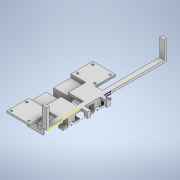
# Autodesk Inventor part: shell 1.0 screw
Saved by Autodesk Inventor 2020.2 (Build 242310000, 310)
## iProperties
Created: 2020-02-28
Part Number: shell 1.0 screw
Material: Generic
Document SubType Name: Modeling
Designer: ColinP
Density: 1 g/cm^3
Appearance: Default
Author: ColinP
Autodesk Inventor part; units mm, degrees
ref_plane "YZ Plane" through (0, 0, 0) normal (1, 0, 0) x (0, 1, 0)
ref_plane "XZ Plane" through (0, 0, 0) normal (0, 1, 0) x (-1, 0, 0)
ref_plane "XY Plane" through (0, 0, 0) normal (0, 0, 1) x (1, 0, 0)
sketch "Sketch1" plane through (0, 0, 0) normal (0, 1, 0) x (-1, 0, 0)
  line L0 (0, 0) -> (8, 0)
  line L1 (8, 0) -> (8, 116.7892)
  line L2 (8, 116.7892) -> (0, 116.7892)
  line L3 (0, 116.7892) -> (0, 0)
  line L4 (8, 0) -> (0, 0)
  line L5 (0, 0) -> (0, -4)
  line L6 (0, -4) -> (8, -4)
  line L7 (8, -4) -> (8, 0)
  line L8 (8, 116.7892) -> (0, 116.7892)
  line L9 (0, 116.7892) -> (0, 120.7892)
  line L10 (0, 120.7892) -> (8, 120.7892)
  line L11 (8, 120.7892) -> (8, 116.7892)
  point P0 (0, 116.7892)
  dimension "d0" = 8
  dimension "d1" = 116.7892
  dimension "d2" = 8
  dimension "d3" = 4
  dimension "d4" = 4
  constraints: 24 end point, 6 parallel, 3 horizontal, 3 perpendicular
  measures "d0" distance of L2.end L1.end
  measures "d1" distance of L1.end L0.end
  measures "d2" distance of L6.end L5.end
  measures "d3" distance of L5.end L4.end
  measures "d4" distance of L8.end L9.end
extrude "Extrusion1" add sketch "Sketch1" along normal blind 4 contours L3 L2 L1 L0
extrude "Extrusion2" add sketch "Sketch1" along normal blind 34 contours L0 L7 L6 L5 | L9 L10 L11 L2
sketch "Sketch2" plane through (0, 0, 0) normal (0, -1, 0) x (1, 0, 0)
  line L0 (0, 0) -> (0, 19.558)
  line L1 (0, 116.7892) -> (0, 0) projected
  line L2 (0, 19.558) -> (0, 35.6705)
  line L3 (0, 35.6705) -> (0, 48.3705)
  line L4 (0, 48.3705) -> (-8, 48.3705)
  line L5 (-8, 0) -> (-8, 116.7892) projected
  line L6 (-8, 19.558) -> (-8, 48.3705)
  line L7 (0, 19.558) -> (-8, 19.558)
  dimension "d9" = 19.558
  dimension "d10" = 16.1125
  dimension "d11" = 12.7
  constraints: 12 end point, 5 point on line, 2 perpendicular, 1 collinear
  measures "d9" distance of L0.start L0.end
  measures "d10" distance of L0.end L2.end
  measures "d11" distance of L2.end L3.end
extrude "Extrusion3" add sketch "Sketch2" along normal blind 25
sketch "Sketch3" plane through (0, 0, -4) normal (1, 0, 0) x (0, 0, -1)
  line L0 (-52.3705, -25) -> (-23.558, -25) projected
  line L1 (-37.9642, -25) -> (-37.9642, -13.8875)
  line L2 (-37.9642, -13.8875) -> (-31.5508, -13.8875)
  line L3 (-31.5508, -13.8875) -> (-44.3778, -13.8875)
  line L4 (-44.3778, -13.8875) -> (-41.1646, -8.3222)
  line L5 (-44.3778, -13.8875) -> (-37.9516, -13.8875) construction
  line L6 (-41.1646, -8.3222) -> (-34.7385, -8.3222)
  line L7 (-34.7385, -8.3222) -> (-31.5253, -13.8875)
  line L8 (-31.5253, -13.8875) -> (-34.7385, -19.4528)
  line L9 (-34.7385, -19.4528) -> (-41.1646, -19.4528)
  line L10 (-41.1646, -19.4528) -> (-44.3778, -13.8875)
  line L11 (-23.558, 0) -> (-23.558, -25) projected
  line L12 (-52.3705, 0) -> (-52.3705, -25) projected
  line L13 (-23.558, -25) -> (-52.3705, -25)
  line L14 (-52.3705, -25) -> (-52.3705, -13.8875)
  line L15 (-52.3705, -13.8875) -> (-23.558, -13.8875)
  line L16 (-23.558, -13.8875) -> (-23.558, -25)
  point P0 (-4, 0)
  point P1 (-23.558, -13.8875)
  point P2 (-31.5253, -13.8875)
  point P3 (-44.3778, -13.8875)
  dimension "d14" = 11.1125
  dimension "d15" = 6.4135
  dimension "d16" = 12.827
  dimension "d17" = 6.4262
  dimension "d18" = 60
  dimension "d19" = 6.4262
  dimension "d20" = 120
  dimension "d21" = 120
  dimension "d22" = 6.4262
  dimension "d23" = 120
  dimension "d24" = 6.4262
  dimension "d25" = 120
  constraints: 28 end point, 5 horizontal, 4 parallel, 2 point on line, 1 equal length, 1 midpoint, 1 perpendicular, 1 vertical
  measures "d14" distance of L1.start L1.end
  measures "d15" distance of L1.end L2.end
  measures "d16" distance of L2.end L3.end
  measures "d17" distance of L3.end L4.end
  measures "d18" angle of L5 L4
  measures "d19" distance of L4.end L6.end
  measures "d20" angle of L4 L6
  measures "d21" angle of L6 L7
  measures "d22" distance of L7.end L8.end
  measures "d23" angle of L7 L8
  measures "d24" distance of L8.end L9.end
  measures "d25" angle of L8 L9
extrude "Extrusion4" cut sketch "Sketch3" against normal blind 25.4
sketch "Sketch4" plane through (0, 0, -4) normal (1, 0, 0) x (0, 0, -1)
  line L0 (0, 0) -> (-23.558, 0) projected
  line L1 (-23.558, 0) -> (-29.558, 0)
  line L2 (-29.558, 0) -> (-29.558, -8.89)
  line L3 (-29.558, -8.89) -> (-23.558, -8.89)
  line L4 (-23.558, -8.89) -> (-23.558, 0)
  line L5 (-52.3705, 0) -> (-52.3705, -13.8875) projected
  line L6 (-52.3705, 0) -> (-46.3761, 0)
  line L7 (-46.3761, 0) -> (-46.3761, -8.89)
  line L8 (-46.3761, -8.89) -> (-52.3705, -8.89)
  line L9 (-52.3705, -8.89) -> (-52.3705, 0)
  point P0 (-4, 0)
  dimension "d28" = 6
  dimension "d29" = 8.89
  dimension "d30" = 5.9944
  dimension "d31" = 8.89
  constraints: 16 end point, 4 parallel, 2 horizontal, 2 perpendicular
  measures "d28" distance of L3.end L2.end
  measures "d29" distance of L2.end L1.end
  measures "d30" distance of L7.end L8.end
  measures "d31" distance of L6.end L7.end
extrude "Extrusion5" cut sketch "Sketch4" against normal blind 25.4
sketch "Sketch6" plane through (0, 0, -4) normal (1, 0, 0) x (0, 0, -1)
  line L0 (-29.558, -8.89) -> (-29.558, 0) projected
  line L1 (-29.558, 0) -> (-31.558, 0)
  line L2 (-31.558, 0) -> (-31.558, -8.89)
  line L3 (-31.558, -8.89) -> (-29.558, -8.89)
  line L4 (-29.558, -8.89) -> (-29.558, 0)
  line L5 (-46.3761, -8.89) -> (-46.3761, 0) projected
  line L6 (-46.3761, 0) -> (-44.3761, 0)
  line L7 (-44.3761, 0) -> (-44.3761, -8.89)
  line L8 (-44.3761, -8.89) -> (-46.3761, -8.89)
  line L9 (-46.3761, -8.89) -> (-46.3761, 0)
  point P0 (-4, 0)
  dimension "d44" = 2
  dimension "d45" = 8.89
  dimension "d46" = 2
  constraints: 16 end point, 4 parallel, 2 horizontal, 2 perpendicular, 1 point on line
  measures "d44" distance of L3.end L2.end
  measures "d45" distance of L2.end L1.end
  measures "d46" distance of L7.end L8.end
extrude "Extrusion6" cut sketch "Sketch6" against normal blind 25.4
sketch "Sketch5" plane through (0, -13.8875, 19.558) normal (0, -1, 0) x (1, 0, 0)
  line L0 (-8, 0) -> (0, 0) projected
  line L1 (-4, 0) -> (-4, 28.8125)
  line L2 (-8, 28.8125) -> (0, 28.8125) projected
  line L3 (-4, 14.4063) -> (-4, 4.4063)
  line L4 (-4, 14.4063) -> (6, 14.4063) construction
  line L5 (-4, 4.4063) -> (-4, 24.4062)
  point P0 (0, -19.558)
  dimension "d34" = 10
  dimension "d35" = 90
  dimension "d36" = 20
  constraints: 8 end point, 3 midpoint, 1 horizontal, 1 perpendicular, 1 point on line, 1 vertical
  measures "d34" distance of L3.start L3.end
  measures "d35" angle of L3 L4
  measures "d36" distance of L3.end L5.end
hole "Hole1" at (-4, -13.8875, 23.9642) at (-4, -13.8875, 43.9642) direction (0, 1, 0) diameter 3.4 depth 4.9975 clearance for "Flat Head Machine Screw" size "M3" standard "Ansi Metric M Profile"
sketch "Sketch14" plane through (0, 4, 0) normal (0, 1, 0) x (1, 0, 0)
  line L0 (-8, -30.7385) -> (-8, -37.1647) projected
  line L1 (0, -30.7385) -> (-8, -30.7385) projected
  line L2 (0, -37.1647) -> (0, -30.7385) projected
  line L3 (0, -37.1647) -> (-8, -37.1647) projected
  line L4 (-8, -33.9515) -> (-8, -17.7115)
  line L5 (-8, -17.7115) -> (-59.53, -17.7116)
  line L6 (-59.53, -17.7116) -> (-59.53, -50.1916)
  line L7 (-59.53, -50.1916) -> (-8, -50.1915)
  line L8 (-8, -50.1915) -> (-8, -17.7115)
  point P0 (0, 0)
  dimension "d78" = 16.24
  dimension "d79" = 51.53
  dimension "d80" = 32.48
  dimension "d81" = 90
  dimension "d82" = 90
  constraints: 10 end point, 2 perpendicular, 1 midpoint
  measures "d78" distance of L4.start L4.end
  measures "d79" distance of L4.end L5.end
  measures "d80" distance of L5.end L6.end
  measures "d81" angle of L6 L5
  measures "d82" angle of L7 L6
extrude "Extrusion11" add sketch "Sketch14" against normal blind 4 contours L0 L8 L7 L6 L5 L4
sketch "Sketch15" plane through (0, 0, 0) normal (0, -1, 0) x (1, 0, 0)
  line L0 (-59.53, 19.7116) -> (-59.53, 17.7116)
  line L1 (-8, 17.7115) -> (-59.53, 17.7116) projected
  line L2 (-59.53, 17.7116) -> (-57.53, 17.7116)
  line L3 (-57.53, 17.7116) -> (-57.53, 19.7116)
  line L4 (-57.53, 19.7116) -> (-59.53, 19.7116)
  line L5 (-59.53, 19.7116) -> (-59.53, 17.7116)
  line L6 (-59.53, 50.1916) -> (-59.53, 17.7116) projected
  line L7 (-59.53, 50.1916) -> (-30.53, 50.1916)
  line L8 (-30.53, 50.1916) -> (-30.53, 48.1916)
  line L9 (-30.53, 48.1916) -> (-59.53, 48.1916)
  line L10 (-59.53, 48.1916) -> (-59.53, 50.1916)
  line L11 (-30.53, 48.1916) -> (-57.53, 48.1916)
  line L12 (-57.53, 48.1916) -> (-57.53, 19.7116)
  line L13 (-57.53, 19.7116) -> (-30.53, 19.7116)
  line L14 (-30.53, 19.7116) -> (-30.53, 48.1916)
  line L15 (-30.53, 19.7116) -> (-57.53, 19.7116)
  line L16 (-57.53, 19.7116) -> (-57.53, 17.7116)
  line L17 (-57.53, 17.7116) -> (-30.53, 17.7116)
  line L18 (-30.53, 17.7116) -> (-30.53, 19.7116)
  line L19 (-8, -4) -> (-8, 17.7116) projected
  line L20 (0, -4) -> (-8, -4) projected
  line L21 (0, 27.558) -> (0, -4) projected
  line L22 (0, 27.558) -> (-8, 27.558) projected
  line L23 (-8, 40.3761) -> (-8, 27.558) projected
  line L24 (0, 40.3761) -> (-8, 40.3761) projected
  line L25 (0, 120.7892) -> (0, 40.3761) projected
  line L26 (-8, 120.7892) -> (0, 120.7892) projected
  line L27 (-8, 50.1915) -> (-8, 120.7892) projected
  line L28 (-8, 50.1915) -> (-59.53, 50.1916) projected
  line L29 (-59.53, 50.1916) -> (-59.53, 17.7116) projected
  line L30 (-59.53, 17.7116) -> (-8, 17.7116) projected
  point P0 (0, 0)
  dimension "d87" = 2
  dimension "d88" = 2
  dimension "d89" = 29
  dimension "d90" = 2
  constraints: 34 end point, 8 parallel, 4 horizontal, 4 perpendicular
  measures "d87" distance of L4.end L3.end
  measures "d88" distance of L3.end L2.end
  measures "d89" distance of L8.end L9.end
  measures "d90" distance of L7.end L8.end
extrude "Extrusion12" add sketch "Sketch15" along normal blind 36 contours L4 L3 L1 L0 | L6 L9 L12 L4 | L13 L18 L1 L3 | L6 L7 L8 L9
sketch "Sketch16" plane through (-30.53, 0, 48.1916) normal (1, 0, 0) x (0, 0, -1)
  line L0 (7.8155, 0) -> (20.6335, 0) projected
  line L1 (14.2245, 0) -> (14.2245, -13.878)
  line L2 (14.2245, -13.878) -> (14.2245, -21.878)
  line L3 (14.2245, -21.878) -> (31.7245, -21.878)
  line L4 (31.7245, -21.878) -> (-3.2755, -21.878)
  line L5 (-3.2755, -21.878) -> (-3.2755, -18.378)
  line L6 (-3.2755, -18.378) -> (-2, -18.378)
  line L7 (-2, 0) -> (-2, -36) projected
  line L8 (-2, -18.378) -> (-7, -18.378)
  line L9 (-7, -18.378) -> (-7, -25.378)
  line L10 (-7, -18.378) -> (0, -18.378) construction
  line L11 (-7, -25.378) -> (-2, -25.378)
  line L12 (-2, -18.378) -> (-2, -25.378)
  line L13 (30.48, 0) -> (30.48, -36) projected
  line L14 (30.48, -25.378) -> (35.48, -25.378)
  line L15 (35.48, -25.378) -> (35.48, -18.378)
  line L16 (35.48, -18.378) -> (30.48, -18.378)
  circle A0 centre (-3.2755, -21.878) radius 1.7
  circle A1 centre (31.7245, -21.878) radius 1.7
  point P0 (48.1916, 0)
  point P1 (-2, -23.0019)
  point P2 (-3.2755, -20.178)
  point P3 (-3.2755, -18.378)
  point P4 (30.48, -20.7199)
  point P5 (30.48, -23.0361)
  point P6 (-2, -20.7541)
  dimension "d93" = 13.878
  dimension "d94" = 8
  dimension "d95" = 180
  dimension "d96" = 17.5
  dimension "d97" = 90
  dimension "d98" = 35
  dimension "d99" = 3.5
  dimension "d100" = 5
  dimension "d101" = 7
  dimension "d102" = 90
  dimension "d103" = 5
  dimension "d104" = 3.4
  dimension "d105" = 3.4
  constraints: 28 end point, 8 perpendicular, 8 point on line, 2 centre point, 2 coincident, 2 vertical, 1 collinear, 1 horizontal, 1 midpoint
  measures "d93" distance of L1.start L1.end
  measures "d94" distance of L1.end L2.end
  measures "d95" angle of L2 L1
  measures "d96" distance of L2.end L3.end
  measures "d97" angle of L3 L2
  measures "d98" distance of L3.end L4.end
  measures "d99" distance of L4.end L5.end
  measures "d100" distance of L6.end L8.end
  measures "d101" distance of L8.end L9.end
  measures "d102" angle of L9 L10
  measures "d103" distance of L14.start L14.end
  measures "d104" diameter of A0
  measures "d105" diameter of A1
extrude "Extrusion13" cut sketch "Sketch16" against normal blind 25.4 contours A1 L13 L3 | L3 L13 A1 | L13 A1 | A0 L7 L4 | L4 L7 A0 | L7 A0 L5 L4 | L4 L5 A0 L7
extrude "Extrusion14" add sketch "Sketch16" against normal blind 6.4262 contours L13 L16 L15 L14 A1 | A0 L5 L6 L7 | L7 L11 L9 L8 L5 A0
sketch "Sketch17" plane through (-59.53, 4, 17.7116) normal (-1, 0, 0) x (0, 0, 1)
  point P0 (-17.7115, -4)
sketch "Sketch18" plane through (-59.53, 4, 17.7116) normal (-1, 0, 0) x (0, 0, 1)
  line L0 (-5, -29.378) -> (0, -29.378) projected
  line L1 (0, -22.378) -> (-5, -22.378) projected
  line L2 (0, -29.378) -> (1, -29.378)
  line L3 (1, -29.378) -> (1, -22.378)
  line L4 (1, -22.378) -> (0, -22.378)
  line L5 (0, -22.378) -> (0, -29.378)
  line L6 (32.48, 0) -> (32.48, -40) projected
  line L7 (32.48, -22.378) -> (31.48, -22.378)
  line L8 (31.48, -22.378) -> (31.48, -29.378)
  line L9 (31.48, -29.378) -> (32.48, -29.378)
  line L10 (32.48, -29.378) -> (32.48, -22.378)
  point P0 (-17.7115, -4)
  dimension "d110" = 1
  dimension "d111" = 1
  constraints: 16 end point, 4 parallel, 2 horizontal, 2 perpendicular, 1 point on line
  measures "d110" distance of L4.end L3.end
  measures "d111" distance of L9.end L8.end
extrude "Extrusion15" cut sketch "Sketch18" against normal up to surface (22.5738 mm away)
sketch "Sketch21" plane through (0, 0, 0) normal (0, -1, 0) x (1, 0, 0)
  line L0 (-8, 48.3705) -> (-8, 40.3761) projected
  line L1 (-8, 48.3705) -> (-8, 93.1705)
  line L2 (-8, 50.1915) -> (-8, 116.7892) projected
  line L3 (0, 116.7892) -> (0, 0) projected
  line L4 (-8, 93.1705) -> (0, 93.1705)
  line L5 (0, 93.1705) -> (0, 64.3669)
  line L6 (0, 64.3669) -> (-8, 64.3669)
  line L7 (-8, 64.3669) -> (-8, 93.1705)
  dimension "d128" = 44.8
  dimension "d129" = 28.8036
  constraints: 10 end point, 2 parallel, 2 point on line, 1 horizontal, 1 perpendicular
  measures "d128" distance of L0.start L1.end
  measures "d129" distance of L4.end L5.end
extrude "Extrusion18" add sketch "Sketch21" along normal blind 25.4
sketch "Sketch22" plane through (0, 0, -4) normal (1, 0, 0) x (0, 0, -1)
  line L0 (-68.3669, -25.4) -> (-97.1705, -25.4) projected
  line L1 (-82.7687, -25.4) -> (-82.7687, 0)
  line L2 (-82.7687, 0) -> (-82.7687, -8.3285)
  line L3 (-52.3705, -8.89) -> (-44.3761, -8.89) projected
  line L4 (-82.7687, -8.3285) -> (-85.9818, -8.3285)
  line L5 (-85.9818, -8.3285) -> (-89.1949, -13.8938)
  line L6 (-82.7687, -8.3285) -> (-79.5556, -8.3285)
  line L7 (-79.5556, -8.3285) -> (-76.3425, -13.8938)
  line L8 (-76.3425, -13.8938) -> (-68.3669, -13.8938)
  line L9 (-68.3669, -13.8938) -> (-97.1705, -13.8938)
  line L10 (-97.1705, 0) -> (-97.1705, -25.4) projected
  line L11 (-97.1705, -13.8938) -> (-97.1705, 0)
  line L12 (-97.1705, 0) -> (-68.3669, 0)
  line L13 (-68.3669, 0) -> (-68.3669, -13.8938)
  line L14 (-68.3669, -25.4) -> (-68.3669, -13.8938)
  point P0 (-4, 0)
  dimension "d132" = 3.2131
  dimension "d133" = 6.4262
  dimension "d134" = 120
  dimension "d135" = 3.2131
  dimension "d136" = 6.4262
  dimension "d137" = 120
  dimension "d141" = 13.8938
  constraints: 24 end point, 4 perpendicular, 2 horizontal, 2 point on line, 2 vertical, 1 midpoint, 1 parallel
  measures "d132" distance of L2.end L4.end
  measures "d133" distance of L4.end L5.end
  measures "d134" angle of L5 L4
  measures "d135" distance of L2.end L6.end
  measures "d136" distance of L6.end L7.end
  measures "d137" angle of L6 L7
  measures "d141" distance of L9.end L10.start
extrude "Extrusion19" cut sketch "Sketch22" against normal blind 25.4 contours L0 L1 L9 L8 L14 | L0 L10 L9 L1 | L9 L5 L4 L1 | L1 L6 L7 L9
sketch "Sketch23" plane through (0, 0, -4) normal (1, 0, 0) x (0, 0, -1)
  line L0 (-44.3761, -8.89) -> (-52.3705, -8.89) projected
  line L1 (-52.3705, -8.89) -> (-68.3669, -8.89)
  line L2 (-68.3669, 0) -> (-68.3669, -13.8938) projected
  line L3 (-68.3669, -8.89) -> (-76.3679, -8.89)
  line L4 (-76.3679, -8.89) -> (-76.3679, 0)
  line L5 (-54.1915, 0) -> (-68.3669, 0) projected
  line L6 (-76.3679, 0) -> (-68.3669, 0)
  line L7 (-68.3669, 0) -> (-68.3669, -8.89)
  line L8 (-97.1705, 0) -> (-97.1705, -13.8938) projected
  line L9 (-97.1705, -8.89) -> (-89.1695, -8.89)
  line L10 (-97.1705, -8.89) -> (-89.1695, -8.89) construction
  line L11 (-89.1695, -8.89) -> (-89.1695, 0)
  line L12 (-89.1695, 0) -> (-97.1705, 0)
  line L13 (-97.1705, 0) -> (-97.1705, -8.89)
  point P0 (-4, 0)
  point P1 (-72.3674, -8.89)
  point P2 (-93.17, -8.89)
  dimension "d140" = 8.001
  dimension "d142" = 8.001
  dimension "d143" = 0
  constraints: 20 end point, 6 perpendicular, 4 horizontal, 2 midpoint, 2 point on line, 1 collinear, 1 horizontal alignment
  measures "d140" distance of L1.end L3.end
  measures "d142" distance of L9.start L9.end
  measures "d143" distance between parallel lines of L9 L10
extrude "Extrusion20" cut sketch "Sketch23" against normal blind 25.4
sketch "Sketch24" plane through (0, -13.8938, 85.1949) normal (0, -1, 0) x (1, 0, 0)
  line L0 (0, -3.2131) -> (-8, -3.2131) projected
  line L1 (0, -9.6393) -> (-8, -9.6393) projected
  line L2 (0, -3.2131) -> (0, -9.6393)
  line L3 (0, -6.4262) -> (-4, -6.4262)
  line L4 (-4, -6.4262) -> (-4, -16.4262)
  line L5 (-4, -16.4262) -> (-4, 3.5738)
  point P0 (0, -85.1949)
  dimension "d146" = 10
  dimension "d147" = 20
  constraints: 8 end point, 1 horizontal, 1 midpoint, 1 perpendicular, 1 point on line, 1 vertical
  measures "d146" distance of L3.end L4.end
  measures "d147" distance of L4.end L5.end
hole "Hole2" at (-4, -13.8938, 68.7687) at (-4, -13.8938, 88.7687) direction (0, 1, 0) diameter 3.4 depth 5.0038 clearance for "Flat Head Machine Screw" size "M3" standard "Ansi Metric M Profile"
sketch "Sketch25" plane through (0, 4, 0) normal (0, 1, 0) x (1, 0, 0)
  line L0 (-8, -75.5556) -> (-8, -81.9818) projected
  line L1 (0, -75.5556) -> (-8, -75.5556) projected
  line L2 (0, -81.9818) -> (0, -75.5556) projected
  line L3 (0, -81.9818) -> (-8, -81.9818) projected
  line L4 (-8, -50.1915) -> (-8, -116.7892) projected
  line L5 (-8, -78.7687) -> (-8, -62.5254)
  line L6 (-8, -62.5254) -> (-8, -95.012)
  line L7 (-8, -95.012) -> (0, -95.012)
  line L8 (0, -95.012) -> (0, -62.5254)
  line L9 (0, -116.7892) -> (0, 0) projected
  line L10 (-8, -62.5254) -> (0, -62.5254)
  line L11 (-8, -62.5254) -> (-59.5366, -62.5254)
  line L12 (-59.5366, -62.5254) -> (-59.5366, -95.012)
  line L13 (-59.5366, -95.012) -> (-8, -95.012)
  dimension "d155" = 16.2433
  dimension "d156" = 32.4866
  dimension "d157" = 51.5366
  constraints: 16 end point, 4 perpendicular, 4 point on line, 1 horizontal
  measures "d155" distance of L5.start L5.end
  measures "d156" distance of L5.end L6.end
  measures "d157" distance of L5.end L11.end
extrude "Extrusion21" add sketch "Sketch25" against normal blind 4 contours L0 L4 L13 L12 L11
sketch "Sketch26" plane through (0, 0, 0) normal (0, -1, 0) x (1, 0, 0)
  line L0 (-59.5366, 95.012) -> (-59.5366, 62.5254) projected
  line L1 (-8, 95.012) -> (-59.5366, 95.012) projected
  line L2 (-59.5366, 62.5254) -> (-30.5298, 62.5254)
  line L3 (-30.5298, 62.5254) -> (-30.5298, 95.012)
  line L4 (-30.5298, 95.012) -> (-59.5366, 95.012)
  line L5 (-59.5366, 95.012) -> (-59.5366, 62.5254)
  line L6 (-30.5298, 62.5254) -> (-32.5298, 62.5254)
  line L7 (-32.5298, 62.5254) -> (-32.5298, 64.5254)
  line L8 (-32.5298, 64.5254) -> (-30.5298, 64.5254)
  line L9 (-30.5298, 64.5254) -> (-30.5298, 62.5254)
  line L10 (-59.5366, 95.012) -> (-57.5366, 95.012)
  line L11 (-57.5366, 95.012) -> (-57.5366, 93.012)
  line L12 (-57.5366, 93.012) -> (-59.5366, 93.012)
  line L13 (-59.5366, 93.012) -> (-59.5366, 95.012)
  line L14 (-57.5366, 93.012) -> (-32.5298, 93.012)
  line L15 (-32.5298, 93.012) -> (-32.5298, 64.5254)
  line L16 (-32.5298, 64.5254) -> (-57.5366, 64.5254)
  line L17 (-57.5366, 64.5254) -> (-57.5366, 93.012)
  line L18 (-32.5298, 93.012) -> (-32.5298, 95.012)
  point P0 (0, 0)
  dimension "d160" = 29.0068
  dimension "d161" = 2
  dimension "d162" = 2
  dimension "d163" = 2
  dimension "d164" = 2
  constraints: 34 end point, 8 parallel, 5 perpendicular, 4 horizontal, 2 point on line
  measures "d160" distance of L4.end L3.end
  measures "d161" distance of L7.end L8.end
  measures "d162" distance of L6.end L7.end
  measures "d163" distance of L11.end L12.end
  measures "d164" distance of L10.end L11.end
extrude "Extrusion22" add sketch "Sketch26" along normal blind 36 contours L1 L11 L12 L0 | L12 L17 L16 L7 L2 L0 | L1 L18 L14 L11
sketch "Sketch27" plane through (-32.5298, 0, 95.012) normal (1, 0, 0) x (0, 0, -1)
  line L0 (39.8205, -18.378) -> (39.8205, -25.378) projected
  line L1 (39.8205, -18.378) -> (32.4866, -18.378)
  line L2 (32.4866, 4) -> (32.4866, -36) projected
  line L3 (32.4866, -18.378) -> (32.4866, -25.378)
  line L4 (32.4866, -25.378) -> (37.4866, -25.378)
  line L5 (37.4866, -25.378) -> (37.4866, -18.378)
  line L6 (0, 4) -> (0, -36) projected
  line L7 (0, -25.378) -> (-5, -25.378)
  line L8 (-5, -25.378) -> (-5, -18.378)
  line L9 (-5, -18.378) -> (0, -18.378)
  circle A0 centre (43.545, -21.878) radius 1.7 projected
  line L10 (43.545, -21.878) -> (16.2433, -21.878)
  line L11 (19.4564, -8.3285) -> (13.0302, -8.3285) projected
  line L12 (16.2433, -21.878) -> (33.7433, -21.878)
  line L13 (33.7433, -21.878) -> (-1.2567, -21.878)
  circle A1 centre (-1.2567, -21.878) radius 1.7
  circle A2 centre (33.7433, -21.878) radius 1.7
  point P0 (95.012, 0)
  point P1 (0, -23.0229)
  point P2 (0, -20.7331)
  point P3 (32.4866, -20.7331)
  point P4 (32.4866, -23.0229)
  dimension "d167" = 7
  dimension "d168" = 5
  dimension "d169" = 5
  dimension "d170" = 17.5
  dimension "d171" = 35
  dimension "d172" = 3.4
  dimension "d173" = 3.4
  constraints: 20 end point, 10 point on line, 3 perpendicular, 2 centre point, 2 coincident, 1 horizontal, 1 parallel, 1 vertical
  measures "d167" distance of L1.end L3.end
  measures "d168" distance of L3.end L4.end
  measures "d169" distance of L7.start L7.end
  measures "d170" distance of L10.end L12.end
  measures "d171" distance of L12.end L13.end
  measures "d172" diameter of A1
  measures "d173" diameter of A2
extrude "Extrusion23" add sketch "Sketch27" against normal blind 5 contours L5 L10 A2 L2 L1 | L5 L4 L2 A2 L10 | L6 A1 L7 L8 L9
extrude "Extrusion24" cut sketch "Sketch27" against normal up to surface (27.0068 mm away) contours L2 L10 A2 | A2 L10 L2 | A1 L13 L6 | L13 A1 L6 picked at (32.4062, -21.2284) picked at (32.4062, -22.5276)
sketch "Sketch28" plane through (-59.5366, 4, 62.5254) normal (-1, 0, 0) x (0, 0, 1)
  line L0 (0, -29.378) -> (-5, -29.378) projected
  line L1 (0, -29.378) -> (1, -29.378)
  line L2 (1, -29.378) -> (1, -22.378)
  line L3 (1, -22.378) -> (0, -22.378)
  line L4 (0, -22.378) -> (0, -29.378)
  line L5 (37.4866, -29.378) -> (32.4866, -29.378) projected
  line L6 (32.4866, -29.378) -> (31.4866, -29.378)
  line L7 (31.4866, -29.378) -> (31.4866, -22.378)
  line L8 (31.4866, -22.378) -> (32.4866, -22.378)
  line L9 (32.4866, -22.378) -> (32.4866, -29.378)
  point P0 (-62.5254, -4)
  dimension "d178" = 1
  dimension "d179" = 1
  constraints: 16 end point, 4 parallel, 2 horizontal, 2 perpendicular, 1 point on line
  measures "d178" distance of L3.end L2.end
  measures "d179" distance of L7.end L8.end
extrude "Extrusion25" cut sketch "Sketch28" against normal up to surface (22.0068 mm away)
sketch "Sketch29" plane through (0, 4, 0) normal (0, 1, 0) x (1, 0, 0)
  line L0 (-8, -17.7115) -> (-59.53, -17.7116) projected
  line L1 (-8, -17.7115) -> (11.05, -17.7115)
  line L2 (11.05, -17.7115) -> (11.05, -7.7115)
  line L3 (11.05, -7.7115) -> (-8, -7.7116)
  line L4 (-8, -7.7116) -> (-8, -17.7115)
  line L5 (11.05, -17.7115) -> (5.97, -17.7115)
  line L6 (5.97, -17.7115) -> (5.97, -7.7115)
  line L7 (5.97, -7.7115) -> (11.05, -7.7115)
  line L8 (11.05, -7.7115) -> (11.05, -17.7115)
  point P0 (0, 0)
  dimension "d182" = 19.05
  dimension "d183" = 10
  dimension "d184" = 5.08
  constraints: 16 end point, 4 parallel, 2 horizontal, 2 perpendicular, 1 point on line
  measures "d182" distance of L3.end L2.end
  measures "d183" distance of L2.end L1.end
  measures "d184" distance of L6.end L7.end
extrude "Extrusion26" add sketch "Sketch29" against normal blind 4 contours L4 L3 L6 L1
extrude "Extrusion27" add sketch "Sketch29" against normal blind 10 contours L6 L3 L2 L1
sketch "Sketch30" plane through (0, 0, 17.7115) normal (0, 0, 1) x (1, 0, 0)
  line L0 (11.05, -6) -> (5.97, -6) projected
  line L1 (8.51, -6) -> (8.51, -4)
  circle A0 centre (8.51, -4) radius 1
  point P0 (0, 0)
  dimension "d189" = 2
  dimension "d190" = 2
  constraints: 2 end point, 1 centre point, 1 coincident, 1 midpoint, 1 vertical
  measures "d189" distance of L1.start L1.end
  measures "d190" diameter of A0
extrude "Extrusion28" add sketch "Sketch30" along normal blind 25.4
sketch "Sketch31" plane through (0, 0, 120.7892) normal (1, 0, 0) x (0, 0, -1)
  line L0 (58.2638, 4) -> (25.7772, 4) projected
  line L1 (25.7772, 0) -> (0, 0) projected
  line L2 (108.8901, 4) -> (98.8901, 4)
  line L3 (98.8901, 4) -> (98.8901, 0)
  line L4 (98.8901, 0) -> (108.8901, 0)
  line L5 (108.8901, 0) -> (108.8901, 4)
  point P0 (120.7892, 0)
  dimension "d193" = 10
  constraints: 8 end point, 2 parallel, 2 point on line, 1 horizontal, 1 perpendicular
  measures "d193" distance of L4.end L3.end
sketch "Sketch32" plane through (0, 34, 0) normal (0, 1, 0) x (1, 0, 0)
  line L0 (0, 4) -> (-8, 4) projected
  line L1 (-8, 4) -> (-8, 0) projected
  line L2 (-8, 0) -> (0, 0) projected
  line L3 (0, 0) -> (0, 4) projected
extrude "Extrusion29" cut sketch "Sketch32" against normal blind 30
sketch "Sketch33" plane through (0, 0, -4) normal (0, 0, -1) x (-1, 0, 0)
  line L0 (8, 4) -> (0, 4) projected
  line L1 (0, 0) -> (0, 4) projected
  line L2 (0, 0) -> (8, 0) projected
  line L3 (8, 0) -> (8, 4) projected
  point P0 (0, 0)
extrude "Extrusion30" add sketch "Sketch33" along normal blind 80.5688
sketch "Sketch34" plane through (0, 4, 0) normal (0, 1, 0) x (1, 0, 0)
  line L0 (0, -7.7116) -> (0, 84.5688) projected
  line L1 (-8, 84.5688) -> (-8, -17.7116) projected
  line L2 (0, 84.5688) -> (-8, 84.5688)
  line L3 (-8, 84.5688) -> (-8, 80.5688)
  line L4 (-8, 80.5688) -> (0, 80.5688)
  line L5 (0, 80.5688) -> (0, 84.5688)
  point P0 (0, 0)
  point P1 (0, 80.5688)
  dimension "d198" = 4
  constraints: 8 end point, 2 parallel, 1 horizontal, 1 perpendicular, 1 point on line
  measures "d198" distance of L3.end L2.end
extrude "Extrusion31" add sketch "Sketch34" along normal blind 30
sketch "Sketch35" plane through (0, 0, 17.7115) normal (0, 0, 1) x (1, 0, 0)
  line L0 (0, 4) -> (11.05, 4) projected
  circle A0 centre (8.51, -4) radius 1 projected
  line L1 (0, 0) -> (0, 4) projected
  line L2 (5.97, 0) -> (0, 0) projected
  line L3 (5.97, 0) -> (5.97, -6) projected
  line L4 (11.05, -6) -> (5.97, -6) projected
  line L5 (11.05, 4) -> (11.05, -6) projected
  line L6 (0, 4) -> (11.05, 4) projected
  point P0 (0, 0)
extrude "Extrusion32" add sketch "Sketch35" along normal blind 11.43 contours L0 L5 L4 L3 L2 L1 | A0
sketch "Sketch36" plane through (0, 0, 120.7892) normal (1, 0, 0) x (0, 0, -1)
  line L0 (70.5976, 4) -> (58.2638, 4) projected
  line L1 (70.5976, 0) -> (58.2638, 0)
  line L2 (58.2638, 0) -> (58.2638, 4)
  line L3 (58.2638, 4) -> (70.5976, 4)
  line L4 (70.5976, 4) -> (70.5976, 0)
  point P0 (120.7892, 0)
  constraints: 8 end point, 2 parallel, 1 horizontal, 1 perpendicular
extrude "Extrusion33" add sketch "Sketch36" along normal up to surface (11.05 mm away)
sketch "Sketch37" plane through (0, 0, 0) normal (0, -1, 0) x (1, 0, 0)
  line L0 (0, 50.1915) -> (11.05, 50.1915) projected
  line L1 (0, 62.5254) -> (11.05, 62.5254) projected
  line L2 (5.525, 50.1915) -> (11.05, 50.1915)
  line L3 (11.05, 50.1915) -> (11.05, 62.5254)
  line L4 (11.05, 62.5254) -> (5.525, 62.5254)
  line L5 (5.525, 62.5254) -> (5.525, 50.1915)
  point P0 (0, 0)
  constraints: 8 end point, 2 parallel, 1 horizontal, 1 midpoint, 1 perpendicular
extrude "Extrusion34" add sketch "Sketch37" along normal up to surface (6 mm away)
sketch "Sketch38" plane through (0, 0, 62.5254) normal (0, 0, 1) x (1, 0, 0)
  circle A0 centre (8.51, -4) radius 1 projected
  point P0 (0, 0)
extrude "Extrusion35" add sketch "Sketch38" along normal blind 25.4
sketch "Sketch41" plane through (11.05, 4, 62.5254) normal (1, 0, 0) x (0, 0, -1)
  line L0 (12.3339, -10) -> (0, -10) projected
  line L1 (12.3339, 0) -> (0, 0) projected
  line L2 (12.3339, -10) -> (6.1669, -10)
  line L3 (6.1669, -10) -> (6.1669, 0)
  line L4 (6.1669, 0) -> (12.3339, 0)
  line L5 (12.3339, 0) -> (12.3339, -10)
  point P0 (62.5254, -4)
  point P1 (6.1669, -10)
  constraints: 8 end point, 2 parallel, 1 horizontal, 1 midpoint, 1 perpendicular
extrude "Extrusion37" cut sketch "Sketch41" against normal up to surface (11.05 mm away)
sketch "Sketch42" plane through (11.05, -6, 7.7115) normal (1, 0, 0) x (0, 0, -1)
  line L0 (-21.43, 10) -> (0, 10) projected
  line L1 (0, 0) -> (-15.7974, 0)
  line L2 (-15.7974, 0) -> (-15.7974, 10)
  line L3 (-15.7974, 10) -> (0, 10)
  line L4 (0, 10) -> (0, 0)
  point P0 (7.7115, 6)
  point P1 (0, 10)
  constraints: 8 end point, 2 parallel, 1 horizontal, 1 perpendicular, 1 point on line
extrude "Extrusion38" cut sketch "Sketch42" against normal up to surface (11.05 mm away)
sketch "Sketch43" plane through (0, -8.89, 93.1705) normal (0, 1, 0) x (1, 0, 0)
  circle A0 centre (-4, 4.4018) radius 1.7 projected
  line L0 (-8, 0) -> (-8, 8.001) projected
  line L1 (0, 0) -> (-8, 0) projected
  line L2 (0, 8.001) -> (0, 0) projected
  line L3 (0, 8.001) -> (-8, 8.001) projected
  circle A1 centre (-4, 24.4018) radius 1.7 projected
  line L4 (-8, 20.8026) -> (-8, 28.8036) projected
  line L5 (0, 20.8026) -> (-8, 20.8026) projected
  line L6 (0, 28.8036) -> (0, 20.8026) projected
  line L7 (-8, 28.8036) -> (0, 28.8036) projected
  circle A2 centre (-4, 49.2063) radius 1.7 projected
  line L8 (-8, 44.8) -> (-8, 52.7944) projected
  line L9 (0, 44.8) -> (-8, 44.8) projected
  line L10 (0, 52.7944) -> (0, 44.8) projected
  line L11 (0, 52.7944) -> (-8, 52.7944) projected
  circle A3 centre (-4, 69.2062) radius 1.7 projected
  line L12 (-8, 65.6125) -> (-8, 73.6125) projected
  line L13 (0, 65.6125) -> (-8, 65.6125) projected
  line L14 (0, 73.6125) -> (0, 65.6125) projected
  line L15 (-8, 73.6125) -> (0, 73.6125) projected
  point P0 (0, 93.1705)
extrude "Extrusion39" cut sketch "Sketch43" against normal blind 1.5 contours L0 L3 L2 L1 | A1 | L4 L7 L6 L5 | L8 L11 L10 L9 | L12 L15 L14 L13
sketch "Sketch44" plane through (0, 4, 0) normal (0, 1, 0) x (1, 0, 0)
  line L0 (-59.5366, -95.012) -> (-20.5366, -95.012)
  line L1 (-20.5366, -95.012) -> (-20.5366, -130.012)
  line L2 (-20.5366, -130.012) -> (-59.5366, -130.012)
  line L3 (-59.5366, -130.012) -> (-59.5366, -95.012)
  line L4 (-59.53, -50.1916) -> (-59.53, -17.7116) projected
  line L5 (-59.53, -17.7116) -> (-20.53, -17.7116)
  line L6 (-20.53, -17.7116) -> (-20.53, 17.2884)
  line L7 (-20.53, 17.2884) -> (-59.53, 17.2884)
  line L8 (-59.53, 17.2884) -> (-59.53, -17.7116)
  point P0 (0, 0)
  dimension "d243" = 39
  dimension "d244" = 35
  dimension "d245" = 39
  dimension "d246" = 35
  constraints: 16 end point, 4 parallel, 2 horizontal, 2 perpendicular
  measures "d243" distance of L1.end L2.end
  measures "d244" distance of L0.end L1.end
  measures "d245" distance of L7.end L6.end
  measures "d246" distance of L6.end L5.end
extrude "Extrusion40" add sketch "Sketch44" against normal blind 3
sketch "Sketch45" plane through (0, 4, 0) normal (0, 1, 0) x (1, 0, 0)
  line L0 (-59.53, 17.2884) -> (-59.53, -50.1916) projected
  line L1 (-59.53, 17.2884) -> (-54.53, 17.2884)
  line L2 (-54.53, 17.2884) -> (-54.53, 12.2884)
  line L3 (-54.53, 12.2884) -> (-59.53, 12.2884)
  line L4 (-59.53, 12.2884) -> (-59.53, 17.2884)
  line L5 (-54.53, 12.2884) -> (-24.83, 12.2884)
  line L6 (-24.83, 12.2884) -> (-24.83, -13.7616)
  line L7 (-24.83, -13.7616) -> (-54.53, -13.7616)
  line L8 (-54.53, -13.7616) -> (-54.53, 12.2884)
  line L9 (-59.5366, -62.5254) -> (-59.5366, -130.012) projected
  line L10 (-59.5366, -130.012) -> (-55.5366, -130.012)
  line L11 (-55.5366, -130.012) -> (-55.5366, -126.012)
  line L12 (-55.5366, -126.012) -> (-59.5366, -126.012)
  line L13 (-59.5366, -126.012) -> (-59.5366, -130.012)
  line L14 (-55.5366, -126.012) -> (-25.8366, -126.012)
  line L15 (-25.8366, -126.012) -> (-25.8366, -99.962)
  line L16 (-25.8366, -99.962) -> (-55.5366, -99.962)
  line L17 (-55.5366, -99.962) -> (-55.5366, -126.012)
  point P0 (0, 0)
  dimension "d249" = 5
  dimension "d250" = 5
  dimension "d251" = 29.7
  dimension "d252" = 26.05
  dimension "d253" = 4
  dimension "d254" = 4
  dimension "d255" = 29.7
  dimension "d256" = 26.05
  constraints: 32 end point, 8 parallel, 4 horizontal, 4 perpendicular
  measures "d249" distance of L2.end L3.end
  measures "d250" distance of L1.end L2.end
  measures "d251" distance of L6.end L7.end
  measures "d252" distance of L5.end L6.end
  measures "d253" distance of L12.end L11.end
  measures "d254" distance of L11.end L10.end
  measures "d255" distance of L16.end L15.end
  measures "d256" distance of L15.end L14.end
hole "Hole4" at (-25.8366, 4, 99.962) at (-55.5366, 4, 99.962) at (-25.8366, 4, 126.012) at (-55.5366, 4, 126.012) at (-24.83, 4, 13.7616) at (-24.83, 4, -12.2884) at (-54.53, 4, -12.2884) at (-54.53, 4, 13.7616) direction (0, -1, 0) diameter 3.4 end through all clearance for "Flat Head Machine Screw" size "M3" standard "Ansi Metric M Profile"
sketch "Sketch46" plane through (0, 0, 0) normal (0, -1, 0) x (1, 0, 0)
  line L0 (-57.53, 19.7116) -> (-57.53, 48.1916) projected
  line L1 (-57.53, 19.7116) -> (-30.5066, 19.7116)
  line L2 (-30.5066, 19.7116) -> (-30.5066, 48.1916)
  line L3 (-30.5066, 48.1916) -> (-57.53, 48.1916)
  line L4 (-57.53, 48.1916) -> (-57.53, 19.7116)
  line L5 (-57.5366, 64.5254) -> (-32.5298, 64.5254) projected
  line L6 (-32.5298, 93.012) -> (-57.5366, 93.012) projected
  line L7 (-57.5366, 64.5254) -> (-32.5298, 64.5254)
  line L8 (-32.5298, 64.5254) -> (-32.5298, 93.012)
  line L9 (-32.5298, 93.012) -> (-57.5366, 93.012)
  line L10 (-57.5366, 93.012) -> (-57.5366, 64.5254)
  point P0 (0, 0)
  constraints: 16 end point, 4 parallel, 2 horizontal, 2 perpendicular
extrude "Extrusion41" add sketch "Sketch46" along normal blind 7.8
sketch "Sketch47" plane through (-59.5366, -36, 62.5254) normal (-1, 0, 0) x (0, 0, 1)
  line L0 (0, 40) -> (0, 17.622) projected
  line L1 (0, 40) -> (30, 40)
  line L2 (30, 40) -> (30, 34.3)
  line L3 (30, 34.3) -> (0, 34.3)
  line L4 (0, 34.3) -> (0, 40)
  line L5 (-79.8138, 40) -> (-12.3338, 40) projected
  line L6 (-12.3338, 40) -> (-42.3313, 40)
  line L7 (-42.3313, 40) -> (-42.3312, 34.3)
  line L8 (-42.3312, 34.3) -> (-12.3338, 34.3)
  line L9 (-12.3338, 34.3) -> (-12.3338, 40)
  point P0 (-62.5254, 36)
  point P1 (0, 34.3)
  dimension "d266" = 30
  dimension "d267" = 5.7
  dimension "d268" = 29.9974
  constraints: 16 end point, 4 parallel, 2 horizontal, 2 perpendicular, 1 point on line
  measures "d266" distance of L2.end L3.end
  measures "d267" distance of L1.end L2.end
  measures "d268" distance of L8.end L7.end
extrude "Extrusion42" cut sketch "Sketch47" against normal blind 25.4
body "Solid1"
